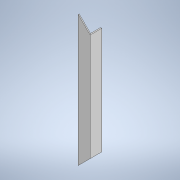
# Autodesk Inventor part: angle4
Saved by Autodesk Inventor 2020.1 (Build 241239000, 239)
## iProperties
Created: 2021-08-04
Part Number: angle4
Material: Generic
Document SubType Name: Modeling
Designer: Caleb
Density: 1 g/cm^3
Appearance: Default
Author: Caleb
Autodesk Inventor part; units mm, degrees
ref_plane "YZ Plane" through (0, 0, 0) normal (1, 0, 0) x (0, 1, 0)
ref_plane "XZ Plane" through (0, 0, 0) normal (0, 1, 0) x (-1, 0, 0)
ref_plane "XY Plane" through (0, 0, 0) normal (0, 0, 1) x (1, 0, 0)
sketch "Sketch1" plane through (0, 0, 0) normal (1, 0, 0) x (0, 1, 0)
  line L0 (-275, 24.5536) -> (275, 24.5536)
  line L1 (275, 24.5536) -> (275, -24.5536)
  line L2 (275, -24.5536) -> (-275, -24.5536)
  line L3 (-275, -24.5536) -> (-275, 24.5536)
  point P0 (0, 0)
  dimension "d18" = 550
  constraints: 8 end point, 2 parallel, 1 horizontal, 1 perpendicular
  measures "d18" distance of L1.end L2.end
extrude "Extrusion1" add sketch "Sketch1" along normal mid plane 50
sketch "Sketch5" plane through (-25, 275, 24.5536) normal (0, 1, 0) x (1, 0, 0)
  line L0 (0, 49.1071) -> (0, 0) projected
  line L1 (0, 49.1071) -> (0, 4.1071)
  line L2 (0, 4.1071) -> (45, 4.1071)
  line L3 (45, 4.1071) -> (45, 49.1071)
  line L4 (0, 49.1071) -> (50, 49.1071) projected
  line L5 (0, 49.1071) -> (45, 49.1071)
  point P0 (25, 24.5536)
  constraints: 8 end point, 3 perpendicular, 2 point on line
extrude "Extrusion5" cut sketch "Sketch5" against normal through all
sketch "Sketch6" plane through (25, 0, 0) normal (1, 0, 0) x (0, 0, -1)
  line L0 (24.5536, -275) -> (24.5536, 275) projected
  line L1 (-20.4464, 275) -> (-20.4464, -275) projected
  line L2 (24.5536, 275) -> (-20.4464, 275)
  line L3 (-20.4464, 275) -> (-20.4464, 225)
  line L4 (-20.4464, 225) -> (24.5536, 225)
  line L5 (24.5536, 225) -> (24.5536, 275)
  line L6 (-24.5536, -275) -> (24.5536, -275) projected
  line L7 (24.5536, -275) -> (-20.4464, -275)
  line L8 (-20.4464, -275) -> (-20.4464, -225)
  line L9 (-20.4464, -225) -> (24.5536, -225)
  line L10 (24.5536, -225) -> (24.5536, -275)
  point P0 (0, 0)
  dimension "d23" = 50
  dimension "d24" = 50
  constraints: 16 end point, 5 perpendicular, 5 point on line
  measures "d23" distance of L1.start L3.end
  measures "d24" distance of L7.end L8.end
extrude "Extrusion6" cut sketch "Sketch6" against normal blind 10 contours L6 L1 L9 L0 | L4 L1 L2 L0
sketch "Sketch7" plane through (-25, -275, 24.5536) normal (0, 0, 1) x (1, 0, 0)
  line L0 (50, 50) -> (50, 500) projected
  line L1 (0, 0) -> (0, 550) projected
  line L2 (50, 500) -> (0, 550)
  line L3 (0, 550) -> (50, 550)
  line L4 (50, 550) -> (50, 500)
  line L5 (50, 50) -> (0, 0)
  line L6 (0, 0) -> (50, 0)
  line L7 (50, 0) -> (50, 50)
  point P0 (25, 275)
  constraints: 12 end point, 5 perpendicular, 2 point on line
extrude "Extrusion7" cut sketch "Sketch7" against normal blind 5 contours L7 L6 L5 | L2 L3 L4
body "Solid1"
